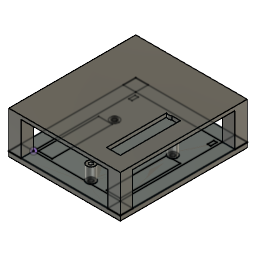
electronics holder (Autodesk Fusion 360 design; units mm, degrees)
part number: 2025-11-18-14-11-44-867
Autodesk Fusion 360 part; units mm, degrees
sketch "Esquisse1" plane through (0, 0, 0) normal (0, 0, 1) x (1, 0, 0)
  line L0 (0, 0) -> (70, 0)
  line L1 (70, 0) -> (70, 82.5)
  line L2 (70, 82.5) -> (0, 82.5)
  line L3 (0, 82.5) -> (0, 0)
  circle A0 centre (43.89, 2.5) radius 1.5
  circle A1 centre (10.87, 54.57) radius 1.5
  circle A2 centre (59.13, 53.3) radius 1.5
  line L4 (-10, -10) -> (80, -10)
  line L5 (80, -10) -> (80, 92.5)
  line L6 (80, 92.5) -> (-10, 92.5)
  line L7 (-10, 92.5) -> (-10, -10)
  line L8 (80, 92.5) -> (70, 92.5)
  line L9 (70, 92.5) -> (70, 82.5)
  line L10 (70, 82.5) -> (80, 82.5)
  line L11 (80, 82.5) -> (80, 92.5)
  line L12 (80, -10) -> (70, -10)
  line L13 (70, -10) -> (70, 0)
  line L14 (70, 0) -> (80, 0)
  line L15 (80, 0) -> (80, -10)
  line L16 (0, 0) -> (-10, 0)
  line L17 (-10, 0) -> (-10, -10)
  line L18 (-10, -10) -> (0, -10)
  line L19 (0, -10) -> (0, 0)
  line L20 (0, 82.5) -> (-10, 82.5)
  line L21 (-10, 82.5) -> (-10, 92.5)
  line L22 (-10, 92.5) -> (0, 92.5)
  line L23 (0, 92.5) -> (0, 82.5)
  line L24 (68, 2) -> (57, 2)
  line L25 (57, 2) -> (57, 50.5)
  line L26 (57, 50.5) -> (68, 50.5)
  line L27 (68, 50.5) -> (68, 2)
  line L28 (2, 50.5) -> (13, 50.5)
  line L29 (13, 50.5) -> (13, 2)
  line L30 (13, 2) -> (2, 2)
  line L31 (2, 2) -> (2, 50.5)
  line L32 (68, 80) -> (65.5, 80)
  line L33 (65.5, 80) -> (65.5, 75)
  line L34 (65.5, 75) -> (68, 75)
  line L35 (68, 75) -> (68, 80)
  line L36 (2, 80) -> (4.5, 80)
  line L37 (4.5, 80) -> (4.5, 75)
  line L38 (4.5, 75) -> (2, 75)
  line L39 (2, 75) -> (2, 80)
  circle A3 centre (10.87, 54.57) radius 3.5
  circle A4 centre (59.13, 53.3) radius 3.5
  circle A5 centre (43.89, 2.5) radius 3.5
  dimension "d1" = 70
  dimension "d2" = 82.5
  dimension "d3" = 3
  dimension "d4" = 26.11
  dimension "d5" = 2.5
  dimension "d6" = 3
  dimension "d7" = 10.87
  dimension "d8" = 27.93
  dimension "d9" = 3
  dimension "d10" = 29.2
  dimension "d12" = 90
  dimension "d13" = 102.5
  dimension "d14" = 10
  dimension "d15" = 10
  dimension "d16" = 10.87
  dimension "d17" = 11
  dimension "d18" = 48.5
  dimension "d19" = 2
  dimension "d20" = 2
  dimension "d21" = 11
  dimension "d22" = 48.5
  dimension "d23" = 2
  dimension "d24" = 2
  dimension "d25" = 2.5
  dimension "d26" = 5
  dimension "d27" = 2.5
  dimension "d28" = 5
  dimension "d29" = 2
  dimension "d30" = 2.5
  dimension "d31" = 2
  dimension "d32" = 2.5
  dimension "d35" = 7
  dimension "d36" = 7
  dimension "d37" = 7
  constraint horizontal L0
  constraint vertical L1
  constraint horizontal L2
  constraint vertical L3
  constraint coincident L0.start L3.end
  constraint horizontal L4
  constraint vertical L5
  constraint horizontal L6
  constraint vertical L7
  constraint horizontal L8
  constraint vertical L9
  constraint horizontal L10
  constraint vertical L11
  constraint horizontal L12
  constraint vertical L13
  constraint horizontal L14
  constraint vertical L15
  constraint horizontal L16
  constraint vertical L17
  constraint horizontal L18
  constraint vertical L19
  constraint horizontal L20
  constraint vertical L21
  constraint horizontal L22
  constraint vertical L23
  constraint horizontal L24
  constraint vertical L25
  constraint horizontal L26
  constraint vertical L27
  constraint horizontal L28
  constraint vertical L29
  constraint horizontal L30
  constraint vertical L31
  constraint horizontal L32
  constraint vertical L33
  constraint horizontal L34
  constraint vertical L35
  constraint horizontal L36
  constraint vertical L37
  constraint horizontal L38
  constraint vertical L39
  constraint concentric A1 A3
  constraint concentric A2 A4
  constraint concentric A0 A5
  measures "d1" distance of L0.start L0.end
  measures "d2" distance of L0.start L2.end
  measures "d3" diameter of A0
  measures "d4" distance of L1 A0.centre
  measures "d5" distance of L0 A0.centre
  measures "d6" diameter of A1
  measures "d7" distance of L3 A1.centre
  measures "d8" distance of L2 A1.centre
  measures "d9" diameter of A2
  measures "d10" distance of L2 A2.centre
  measures "d12" distance of L4.start L4.end
  measures "d13" distance of L4.start L6.end
  measures "d14" distance of L1 L5
  measures "d15" distance of L0 L4
  measures "d16" distance of L1 A2.centre
  measures "d17" distance of L24.start L24.end
  measures "d18" distance of L24.start L26.end
  measures "d19" distance of L1 L27
  measures "d20" distance of L0 L24
  measures "d21" distance of L28.start L28.end
  measures "d22" distance of L28.start L30.end
  measures "d23" distance of L3 L31
  measures "d24" distance of L0 L30
  measures "d25" distance of L32.start L32.end
  measures "d26" distance of L32.start L34.end
  measures "d27" distance of L36.start L36.end
  measures "d28" distance of L36.start L38.end
  measures "d29" distance of L1 L35
  measures "d30" distance of L2 L32
  measures "d31" distance of L3 L39
  measures "d32" distance of L2 L36
  measures "d35" diameter of A3
  measures "d36" diameter of A4
  measures "d37" diameter of A5
extrude "Extrusion1" add sketch "Esquisse1" against normal blind 4 contours L0 L1 L2 L3 A5 | L3 L7 L16 L20 | L4 L7 L16 L17 L18 L19 | L0 L4 L13 L19 A5 | L0 A5 | L0 A5 | L2 L6 L9 L23 | L6 L7 L20 L21 L22 L23 | L1 L5 L10 L14 | L5 L6 L8 L9 L10 L11 | L4 L5 L12 L13 L14 L15 | A0 | A1 | A2 | L24 L25 L26 L27 A4 | L26 A4 | L26 A4 | L28 L29 L30 L31 | L32 L33 L34 L35 | L36 L37 L38 L39 | A3
extrude "Extrusion2" add sketch "Esquisse1" along normal blind 12 contours L0 A5 | L0 A5 | L26 A4 | L26 A4 | A3
extrude "Extrusion3" add sketch "Esquisse1" along normal blind 27 contours L4 L7 L16 L17 L18 L19 | L6 L7 L20 L21 L22 L23 | L5 L6 L8 L9 L10 L11 | L4 L5 L12 L13 L14 L15
sketch "Esquisse3" plane through (0, 0, 27) normal (0, 0, 1) x (-1, 0, 0)
  line L0 (-80, 0) -> (-70, 0)
  line L1 (-70, 0) -> (-70, 10)
  line L2 (-70, 10) -> (-80, 10)
  line L3 (-80, 10) -> (-80, 0)
  line L4 (10, 10) -> (-80, 10)
  line L5 (-80, 10) -> (-80, -92.5)
  line L6 (-80, -92.5) -> (10, -92.5)
  line L7 (10, -92.5) -> (10, 10)
  dimension "d42" = 90
  dimension "d43" = 102.5
  constraint horizontal L4
  constraint vertical L5
  constraint horizontal L6
  constraint vertical L7
  measures "d42" distance of L4.start L2.end
  measures "d43" distance of L4.start L6.end
extrude "Extrusion4" add sketch "Esquisse3" along normal blind 3
extrude "Extrusion5" cut sketch "Esquisse1" along normal blind 40 contours L24 L25 L26 L27 A4
